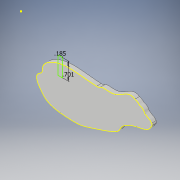
# Autodesk Inventor part: Idea 1
Saved by Autodesk Inventor 2019 (Build 230136000, 136)
## iProperties
Created: 2020-02-12
Part Number: Idea 1
Material: Generic
Document SubType Name: Modeling
Designer: student
Density: 1 g/cm^3
Appearance: Default
Author: student
Autodesk Inventor part; units mm, degrees
ref_plane "YZ Plane" through (0, 0, 0) normal (1, 0, 0) x (0, 1, 0)
ref_plane "XZ Plane" through (0, 0, 0) normal (0, 1, 0) x (-1, 0, 0)
ref_plane "XY Plane" through (0, 0, 0) normal (0, 0, 1) x (1, 0, 0)
sketch "Sketch1" plane through (0, 0, 0) normal (0, 0, 1) x (1, 0, 0)
  line L0 (0, 0) -> (155.2665, 0) construction
  line L1 (155.2665, 0) -> (155.2665, -114.3) construction
  line L2 (155.2665, -114.3) -> (0, -114.3) construction
  line L3 (0, -114.3) -> (0, 0) construction
  spline S0 degree 4 poles (134.4539, -32.6713) (131.6853, -33.0878) (132.3031, -30.1405) (128.7299, -29.0975) (127.9668, -28.7051) (126.7728, -27.595) (125.6869, -27.2229) (124.9703, -26.2256) (124.3627, -24.5047) (123.2609, -23.8545) (121.3724, -22.3115) (119.5472, -22.5506) (118.003, -19.4903) (115.6045, -19.7544) (115.467, -19.3607) knots 0 0 0 0 0 0.211272 0.279618 0.340923 0.399481 0.463887 0.529149 0.59955 0.671433 0.746231 0.826094 1 1 1 1 1
  spline S1 degree 4 poles (115.467, -19.3607) (111.7782, -17.2271) (107.2795, -17.1265) (96.8854, -27.8205) (86.2023, -25.6779) (81.9362, -24.5341) (79.1072, -27.5068) knots 0 0 0 0 0 0.4241 0.599988 1 1 1 1 1
  spline S2 degree 4 poles (79.1072, -27.5068) (53.6175, -26.4047) (45.6753, -20.7652) (16.9609, -31.6927) (23.2196, -43.97) (14.9288, -45.4544) (15.4947, -53.843) (21.2835, -59.899) (25.921, -68.365) (50.4457, -70.2504) (62.1123, -70.1182) (70.1229, -66.5936) (104.0521, -56.6583) (97.2829, -51.1854) (117.6542, -39.7037) (132.2393, -42.2984) (131.1827, -33.5601) (134.4539, -32.6713) knots 0 0 0 0 0 0.195252 0.245812 0.288455 0.330098 0.375992 0.432811 0.494694 0.56024 0.635097 0.699289 0.764609 0.830681 0.884385 1 1 1 1 1
  point P0 (131.7696, -31.3844)
  point P1 (129.9872, -29.6001)
  point P2 (128.4981, -28.932)
  point P3 (127.8596, -28.5585)
  point P4 (126.8072, -27.7466)
  point P5 (125.8037, -27.1289)
  point P6 (125.0665, -26.2208)
  point P7 (124.3033, -24.7785)
  point P8 (123.2261, -23.7723)
  point P9 (121.445, -22.6427)
  point P10 (120.1261, -22.1449)
  point P11 (118.4173, -20.7488)
  point P12 (116.1791, -19.6745)
  point P13 (110.3408, -18.0275)
  point P14 (104.329, -20.3615)
  point P15 (96.1307, -24.796)
  point P16 (88.8376, -25.7335)
  point P17 (83.4118, -25.4981)
  point P18 (43.4642, -25.5282)
  point P19 (26.8269, -31.4039)
  point P20 (21.6011, -38.8087)
  point P21 (20.7479, -43.1813)
  point P22 (16.9085, -46.3808)
  point P23 (16.0553, -52.0332)
  point P24 (19.8947, -58.7521)
  point P25 (26.6136, -65.471)
  point P26 (48.5834, -69.8436)
  point P27 (61.168, -69.417)
  point P28 (73.7526, -65.791)
  point P29 (98.8152, -55.3393)
  point P30 (101.5881, -50.86)
  point P31 (114.0661, -43.5012)
  point P32 (127.9154, -39.6619)
  point P33 (131.7869, -35.5025)
  dimension "d5" = 114.3
  constraints: 1 vertical alignment, 42 other
  measures "d5" distance between parallel lines of L2 L0
extrude "Extrusion1" add sketch "Sketch1" against normal blind 4.699
fillet "Fillet1" radius 1.7145 1 edges at (134.4539, -32.6713, -2.3495)
fillet "Fillet2" radius 6.35 1 edges at (79.1072, -27.5068, -2.3495)
sketch "Sketch2" plane through (0, 0, 0) normal (0, 0, 1) x (1, 0, 0)
  line L0 (37.3888, -19.4804) -> (42.0878, -19.4804)
  line L1 (42.0878, -19.4804) -> (42.0878, -37.289)
  line L2 (42.0878, -37.289) -> (37.3888, -37.289)
  line L3 (37.3888, -37.289) -> (37.3888, -19.4804)
  point P0 (0, 0)
  point P1 (132.5477, -34.2569)
  point P2 (132.3428, -32.092)
  point P3 (115.467, -19.3607)
  point P4 (80.4128, -26.4228)
  point P5 (76.6839, -27.3877)
  dimension "d49" = 4.699
  dimension "d50" = 17.8086
  constraints: 8 end point, 2 parallel, 1 horizontal, 1 perpendicular, 5 other
  measures "d49" distance of L0.start L0.end
  measures "d50" distance of L0.end L1.end
body "Solid1"
